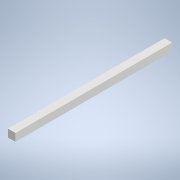
# Autodesk Inventor part: Gantry Brace
Saved by Autodesk Inventor 2022.3 (Build 263350000, 350)
## iProperties
Created: 2022-06-13
Part Number: Gantry Brace
Material: Generic
Document SubType Name: Modeling
Designer: Robert Nies
Density: 1 g/cm^3
Appearance: Default
Author: Robert Nies
Autodesk Inventor part; units mm, degrees
ref_plane "YZ Plane" through (0, 0, 0) normal (1, 0, 0) x (0, 1, 0)
ref_plane "XZ Plane" through (0, 0, 0) normal (0, 1, 0) x (-1, 0, 0)
ref_plane "XY Plane" through (0, 0, 0) normal (0, 0, 1) x (1, 0, 0)
sketch "Sketch1" plane through (0, 0, 0) normal (0, 0, 1) x (1, 0, 0)
  line L0 (0, 0) -> (38.1, 0)
  line L1 (38.1, 0) -> (38.1, -38.1)
  line L2 (38.1, -38.1) -> (0, -38.1)
  line L3 (0, -38.1) -> (0, 0)
  dimension "d0" = 38.1
  dimension "d1" = 38.1
  constraints: 8 end point, 2 parallel, 1 horizontal, 1 perpendicular
  measures "d0" distance of L1.end L2.end
  measures "d1" distance of L0.end L1.end
extrude "Extrusion1" add sketch "Sketch1" along normal blind 787.4
body "Solid1"
